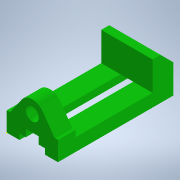
# Autodesk Inventor part: Pieza2 Base
Saved by Autodesk Inventor 2021 (Build 250183000, 183)
## iProperties
Created: 2020-10-13
Part Number: Pieza2 Base
Material: Hierro, fundido
Document SubType Name: Modeling
Designer: aleja
Density: 7.15 g/cm^3
Appearance: Light Red
Author: aleja
Autodesk Inventor part; units mm, degrees
ref_plane "YZ Plane" through (0, 0, 0) normal (1, 0, 0) x (0, 1, 0)
ref_plane "XZ Plane" through (0, 0, 0) normal (0, 1, 0) x (-1, 0, 0)
ref_plane "XY Plane" through (0, 0, 0) normal (0, 0, 1) x (1, 0, 0)
sketch "Boceto1" plane through (0, 0, 0) normal (0, 0, 1) x (1, 0, 0)
  line L0 (64, 24) -> (64, 0)
  line L1 (0, 0) -> (0, 24)
  line L2 (0, 0) -> (0, 24) construction
  line L3 (40, 7) -> (40, 16)
  line L4 (64, 0) -> (64, 24)
  line L5 (0, 24) -> (0, 0)
  line L6 (64, 0) -> (64, 16)
  line L7 (40, 16) -> (24, 16)
  line L8 (0, 16) -> (0, 0)
  line L9 (24, 16) -> (40, 16)
  line L10 (64, 16) -> (64, 7)
  line L11 (0, 7) -> (0, 16)
  line L12 (48, 0) -> (48, 7)
  line L13 (16, 7) -> (16, 0)
  line L14 (24, 16) -> (24, 7)
  line L15 (48, 7) -> (40, 7)
  line L16 (24, 7) -> (16, 7)
  arc A0 (45.1449, 45.122) -> (18.8863, 45.1669) centre (32, 36) ccw
  circle A1 centre (32, 36) radius 8
  line L17 (64, 24) -> (59.8026, 24)
  line L18 (4.09, 24) -> (0, 24)
  line L19 (64, 0) -> (48, 0)
  line L20 (16, 0) -> (0, 0)
  line L21 (0, 0) -> (16, 0)
  line L22 (48, 0) -> (60.5696, 0)
  line L23 (0, 0) -> (16, 0)
  line L24 (48, 0) -> (64, 0)
  line L25 (0, 0) -> (16, 0)
  line L26 (48, 0) -> (64, 0)
  line L27 (4.09, 24) -> (18.8863, 45.1669)
  line L28 (45.1449, 45.122) -> (59.8026, 24)
  line L29 (16, 0) -> (48, 0)
  line L30 (0, 0) -> (64, 0)
  line L31 (64, 0) -> (64, 24)
  line L32 (32.0546, 51.9999) -> (31.9454, 51.9999)
  line L33 (0, 24) -> (0, 0)
  line L34 (0, 0) -> (64, 0)
  line L35 (64, 0) -> (64, 53.4326)
  line L36 (64, 53.4326) -> (0, 53.4326)
  line L37 (0, 53.4326) -> (0, 0)
  circle A2 centre (32, 36) radius 8
  point P0 (30.2848, 0)
  dimension "d6" = 24
  dimension "d9" = 32
  dimension "d10" = 16
  dimension "d11" = 9
  constraints: 76 end point, 14 parallel, 12 horizontal, 7 perpendicular, 5 point on circle, 3 centre point, 3 point on line, 2 coincident, 2 tangent, 1 collinear, 1 concentric, 1 vertical
  measures "d6" distance of L0.start L4.start
  measures "d9" distance between parallel lines of L13 L12
  measures "d10" distance between parallel lines of L14 L3
  measures "d11" distance of L3.start L3.end
sketch "Boceto2" plane through (0, 0, 0) normal (1, 0, 0) x (0, 1, 0)
  point P0 (0, 0)
sketch "Boceto3" plane through (0, 0, 0) normal (1, 0, 0) x (0, 1, 0)
  point P0 (0, 0)
sketch "Boceto4" plane through (0, 0, 0) normal (1, 0, 0) x (0, 1, 0)
  line L0 (0, 0) -> (0, -144)
  line L1 (0, -144) -> (36, -144)
  line L2 (0, -144) -> (16, -144)
  line L3 (16, -118) -> (16, -22)
  line L4 (16, 0) -> (0, 0)
  line L5 (0, 0) -> (0, -144)
  line L6 (36, -144) -> (16, -144)
  line L7 (16, -118) -> (52, -118)
  line L8 (52, -118) -> (52, -128)
  line L9 (36, -144) -> (52, -128)
  line L10 (52, 0) -> (16, 0)
  line L11 (16, -22) -> (52, -22)
  line L12 (52, -22) -> (52, 0)
  line L13 (52, -128) -> (52, -118)
  line L14 (52, -22) -> (52, 0)
  dimension "d15" = 144
  dimension "d17" = 16
  dimension "d22" = 22
  constraints: 30 end point, 4 parallel, 4 perpendicular, 3 horizontal, 1 collinear, 1 vertical
  measures "d15" distance of L0.start L0.end
  measures "d17" distance between parallel lines of L0 L3
  measures "d22" distance between parallel lines of L10 L11
extrude "Extrusión1" add sketch "Boceto4" along normal blind 64
extrude "Extrusión3" cut sketch "Boceto1" against normal blind 100 contours L17 L28 A0 L27 L18 L37 L36 L35
extrude "Extrusión4" cut sketch "Boceto1" against normal blind 100 contours A1
extrude "Extrusión5" cut sketch "Boceto1" against normal blind 144 contours L29 L13 L16 L14 L7 L3 L15 L12
fillet "Empalme1" radius 3 2 edges at (59.8026, 24, -11) (4.09, 24, -11)
